Autodesk Fusion 360 part; units mm, degrees
note: some values were not read from the file. Set by a fixed rule: which face or edge a step refers to.
(part 2 of 2)
sketch "lid base (2)" plane through (0, 0, 0) normal (0, 0, 1) x (1, 0, 0) in component "lid, vented"
  line L0 (33.4, 49.8) -> (33.4, -1.75) construction
  line L1 (35, 49.8) -> (33.4, 49.8)
  line L2 (33.4, 55.6) -> (35, 55.6) construction
  line L3 (35, 55.6) -> (35, 66.15)
  line L4 (35, 49.8) -> (35, -1.75)
  line L5 (35, 49.8) -> (35, 55.6)
  line L6 (35, 66) -> (-9.2, 66)
  line L7 (-9.2, -1.6) -> (35, -1.6)
  line L8 (33.25, 49.8) -> (33.25, 0)
  line L9 (-7.45, 64.25) -> (33.25, 64.25)
  line L10 (33.25, 64.25) -> (33.25, 55.6)
  line L11 (-6.65, 0) -> (-6.65, 63.45)
  line L12 (32.45, 63.45) -> (32.45, 55.6)
  line L13 (35, 55.45) -> (32.45, 55.45)
  line L14 (32.45, 55.45) -> (32.45, 55.6)
  line L15 (33.25, 55.6) -> (33.25, 55.45)
  line L16 (33.4, -1.75) -> (-7.6, -1.75) construction
  line L17 (-7.6, 0) -> (33.4, 0)
  line L18 (-7.45, 0) -> (-7.45, -1.6)
  line L19 (33.25, 0) -> (33.25, -1.6)
  line L20 (31, 41) -> (33.4, 41)
  line L21 (35, 49.95) -> (32.45, 49.95)
  line L22 (32.45, 55.45) -> (32.45, 49.95)
  line L23 (32.45, 49.95) -> (32.45, 0)
  line L24 (32.45, 63.45) -> (32.45, 64.25)
  line L25 (-6.65, 63.45) -> (-6.65, 64.25)
  line L26 (33.25, 64.25) -> (33.25, 66)
  line L27 (33.25, 49.8) -> (33.25, 49.95)
  line L28 (-7.45, 64.25) -> (-7.45, 66)
  line L29 (-7.6, -1.75) -> (-9.2, -1.75) construction
  line L30 (-7.6, 66.15) -> (-9.2, 66.15) construction
  line L31 (-9.2, 55.6) -> (-9.2, 66.15)
  line L32 (-7.6, -1.75) -> (-7.6, 49.8) construction
  line L33 (33.4, 49.8) -> (33.4, -1.75) construction
  line L34 (33.4, 66.15) -> (33.4, 55.6) construction
  line L35 (35, -1.75) -> (33.4, -1.75) construction
  line L36 (35, 66.15) -> (33.4, 66.15) construction
  line L37 (0, 41) -> (-7.6, 41)
  line L38 (12.9, 64.25) -> (12.9, 0) construction
  line L39 (-9.2, 55.45) -> (-6.65, 55.45)
  line L40 (-9.2, 49.8) -> (-9.2, 55.6)
  line L41 (-9.2, 49.95) -> (-6.65, 49.95)
  line L42 (-7.45, 0) -> (-7.45, 49.95)
  line L43 (-7.45, 55.45) -> (-7.45, 64.25)
  line L44 (-9.2, -1.75) -> (-9.2, 49.8)
  line L45 (-7.6, 55.6) -> (-7.6, 66.15)
  dimension "d193_1" = 0.15
  dimension "d194_1" = 0.8
  dimension "d199_1" = 0.15
  dimension "d200_1" = 0.15
  dimension "d206_1" = 0.15
  dimension "d207_1" = 0.8
  dimension "d210_1" = 0.15
  constraint coincident L1.start L4.start
  constraint coincident L2.end L3.start
  constraint coincident L3 L6.start
  constraint coincident L4 L7.end
  constraint perpendicular L4 L7
  constraint coincident L5 L13.start
  constraint perpendicular L5 L13
  constraint perpendicular L13 L14
  constraint coincident L13 L15.end
  constraint perpendicular L13 L15
  constraint parallel L0 L8
  constraint collinear L8 L10
  constraint coincident L18.start L17
  constraint coincident L11.start L17
  constraint coincident L8.end L17
  constraint coincident L7 L18.end
  constraint perpendicular L7 L18
  constraint coincident L7 L19.end
  constraint perpendicular L7 L19
  constraint coincident L5 L21.start
  constraint perpendicular L14 L21
  constraint perpendicular L21 L22
  constraint coincident L17 L23.end
  constraint perpendicular L17 L23
  constraint coincident L9 L24.end
  constraint perpendicular L9 L24
  constraint coincident L9 L25.end
  constraint perpendicular L9 L25
  constraint coincident L6 L26.end
  constraint perpendicular L6 L26
  constraint coincident L21 L27.end
  constraint perpendicular L21 L27
  constraint coincident L6 L28.end
  constraint perpendicular L6 L28
  constraint midpoint L9 L38.start
  constraint midpoint L17 L38.end
  constraint perpendicular L17 L38
  constraint symmetric L1.start L38 L40.start
  constraint symmetric L2.end L38 L31.start
  constraint symmetric L13.start L38 L39.start
  constraint symmetric L13.end L38 L39.end
  constraint symmetric L21.start L38 L41.start
  constraint symmetric L21.end L38 L41.end
  constraint coincident L41 L42.end
  constraint coincident L39 L43.start
  constraint collinear L12 L24
  constraint perpendicular L39 L43
  measures "d193_1" distance of L7 L16
  measures "d194_1" distance of L11 L42
  measures "d199_1" distance of L0 L8
  measures "d200_1" distance of L2 L13
  measures "d206_1" distance of L1 L21
  measures "d207_1" distance of L8 L23
  measures "d210_1" distance of L6 L30
extrude "Extrude1'''" add sketch "lid base (2)" along normal blind 1.6 separate body makes body 3 in component "lid, vented"
extrude "Extrude2''" add sketch "lid base (2)" against normal blind 1.6 contours L5 L13 L21 L22 | L6 L9 L26 L28 | L9 L10 L12 L13 L14 L15 L24 | L8 L20 L21 L23 L27 | L9 L11 L25 L39 L43 | L11 L39 L40 L41 | L7 L17 L18 L19 | L11 L37 L41 L42 bodies 3 in component "lid, vented"
chamfer "Chamfer1''" distance 0.2 angle 45 1 edges at (35, 52.7, -1.6) on bodies 3 in component "lid, vented"
sketch "nubs (2)" plane through (0, 66, 0) normal (0, 1, 0) x (-1, 0, 0) in component "lid, vented"
  line L0 (-35, 0) -> (-33.25, 0)
  line L1 (-33.25, 0) -> (-33.25, -1.6)
  line L2 (-33.25, -1.6) -> (7.45, -1.6)
  line L3 (7.45, -1.6) -> (7.45, 0)
  line L4 (7.45, 0) -> (9.2, 0)
  line L5 (9.2, 0) -> (9.2, 1.6)
  line L6 (9.2, 1.6) -> (-35, 1.6)
  line L7 (-35, 1.6) -> (-35, 0)
  line L8 (-33.25, 0) -> (7.45, 0) construction
  line L9 (-27.65, -0.3) -> (-29.25, -0.3)
  line L10 (-29.25, -0.3) -> (-29.25, 0.3)
  line L11 (-29.25, 0.3) -> (-27.65, 0.3)
  line L12 (-27.65, 0.3) -> (-27.65, -0.3)
  line L13 (-27.65, -0.3) -> (-29.25, 0.3) construction
  line L14 (-29.25, -0.3) -> (-27.65, 0.3) construction
  line L15 (-12.9, 1.6) -> (-12.9, -1.6) construction
  line L16 (3.45, 0.3) -> (1.85, 0.3)
  line L17 (3.45, -0.3) -> (3.45, 0.3)
  line L18 (1.85, -0.3) -> (3.45, -0.3)
  line L19 (1.85, 0.3) -> (1.85, -0.3)
  point P0 (-28.45, 0)
  dimension "d213_1" = 1.6
  dimension "d214_1" = 0.6
  dimension "d215_1" = 4
  constraint coincident L0.end L1.start
  constraint coincident L3.end L4.start
  constraint horizontal L9
  constraint perpendicular L9 L10
  constraint parallel L9 L11
  constraint parallel L10 L12
  constraint coincident L13 P0
  constraint coincident L14 P0
  constraint coincident L8 P0
  constraint midpoint L6 L15.start
  constraint midpoint L2 L15.end
  constraint symmetric L9.start L15 L18.start
  constraint symmetric L9.end L15 L17.start
  constraint symmetric L10.end L15 L16.start
  constraint symmetric L11.end L15 L16.end
  measures "d213_1" distance of L10.end L11.end
  measures "d214_1" distance of L9.end L10.end
  measures "d215_1" distance of L1 L10
extrude "Extrude3''" add sketch "nubs (2)" along normal blind 0.35 contours L9 L10 L11 L12 | L16 L17 L18 L19 bodies 3 in component "lid, vented"
mirror "Mirror1''" about plane through (31.2, 32.2, -13) normal (0, 1, 0) of "Extrude3''" in component "lid, vented"
fillet "Fillet1''" radius 0.25 4 faces at (28.1833, 66.35, -0.1) (-2.3833, 66.35, -0.1) (28.1833, -1.95, -0.1) (-2.3833, -1.95, -0.1) on bodies 3 in component "lid, vented"
sketch "vent" plane through (0, 0, 0) normal (0, 0, -1) x (1, 0, 0) in component "lid, vented"
  line L0 (33.25, -49.95) -> (35, -49.95)
  line L1 (35, -49.95) -> (35, 1.6)
  line L2 (35, 1.6) -> (33.25, 1.6)
  line L3 (33.25, 1.6) -> (33.25, 0)
  line L4 (33.25, 0) -> (-7.45, 0)
  line L5 (-7.45, 0) -> (-7.45, 1.6)
  line L6 (-7.45, 1.6) -> (-9.2, 1.6)
  line L7 (-9.2, 1.6) -> (-9.2, -49.95)
  line L8 (-9.2, -49.95) -> (-7.45, -49.95)
  line L9 (-7.45, -49.95) -> (-7.45, -41)
  line L10 (-7.45, -41) -> (-6.65, -41)
  line L11 (-6.65, -41) -> (-6.65, -64.25)
  line L12 (-6.65, -64.25) -> (32.45, -64.25)
  line L13 (32.45, -64.25) -> (32.45, -41)
  line L14 (32.45, -41) -> (33.25, -41)
  line L15 (33.25, -41) -> (33.25, -49.95)
  line L16 (-6.65, -61.25) -> (21.85, -61.25) construction
  line L17 (21.85, -61.25) -> (21.85, -43.85) construction
  line L18 (21.85, -43.85) -> (-6.65, -43.85) construction
  line L19 (-6.65, -43.85) -> (-6.65, -61.25) construction
  line L20 (20.85, -44.85) -> (-5.65, -44.85) construction
  line L21 (-5.65, -44.85) -> (-5.65, -60.25) construction
  line L22 (-5.65, -60.25) -> (20.85, -60.25) construction
  line L23 (20.85, -60.25) -> (20.85, -44.85) construction
  line L24 (3.6, -44.85) -> (11.6, -60.25) construction
  line L25 (7.6, -60.25) -> (7.6, -44.85) construction
  line L26 (-12.4, -44.85) -> (-4.4, -60.25) construction
  line L27 (-8.4, -44.85) -> (-0.4, -60.25) construction
  line L28 (-4.4, -44.85) -> (3.6, -60.25) construction
  line L29 (-0.4, -44.85) -> (7.6, -60.25) construction
  line L30 (7.6, -44.85) -> (15.6, -60.25) construction
  line L31 (11.6, -44.85) -> (19.6, -60.25) construction
  line L32 (15.6, -44.85) -> (23.6, -60.25) construction
  line L33 (19.6, -44.85) -> (27.6, -60.25) construction
  line L34 (-5.9911, -58.9225) -> (-5.4787, -59.9089)
  arc A0 (-5.4787, -59.9089) -> (-4.0589, -59.1713) centre (-4.7688, -59.5401) ccw
  line L35 (-4.0589, -59.1713) -> (-4.5713, -58.1849)
  arc A1 (-4.5713, -58.1849) -> (-5.9911, -58.9225) centre (-5.2812, -58.5537) ccw
  line L36 (-5.65, -57.8438) -> (-4.4, -60.25) construction
  line L37 (-5.9911, -51.2225) -> (-1.4787, -59.9089)
  arc A2 (-1.4787, -59.9089) -> (-0.0589, -59.1713) centre (-0.7688, -59.5401) ccw
  line L38 (-0.0589, -59.1713) -> (-4.5713, -50.4849)
  arc A3 (-4.5713, -50.4849) -> (-5.9911, -51.2225) centre (-5.2812, -50.8537) ccw
  line L39 (-5.65, -50.1438) -> (-0.4, -60.25) construction
  line L40 (-4.7411, -45.9287) -> (2.5213, -59.9089)
  arc A4 (2.5213, -59.9089) -> (3.9411, -59.1713) centre (3.2312, -59.5401) ccw
  line L41 (3.9411, -59.1713) -> (-3.3213, -45.1911)
  arc A5 (-3.3213, -45.1911) -> (-4.7411, -45.9287) centre (-4.0312, -45.5599) ccw
  line L42 (-4.4, -44.85) -> (3.6, -60.25) construction
  line L43 (-0.7411, -45.9287) -> (6.5213, -59.9089)
  arc A6 (6.5213, -59.9089) -> (7.9411, -59.1713) centre (7.2312, -59.5401) ccw
  line L44 (7.9411, -59.1713) -> (0.6787, -45.1911)
  arc A7 (0.6787, -45.1911) -> (-0.7411, -45.9287) centre (-0.0312, -45.5599) ccw
  line L45 (-0.4, -44.85) -> (7.6, -60.25) construction
  line L46 (3.2589, -45.9287) -> (10.5213, -59.9089)
  arc A8 (10.5213, -59.9089) -> (11.9411, -59.1713) centre (11.2312, -59.5401) ccw
  line L47 (11.9411, -59.1713) -> (4.6787, -45.1911)
  arc A9 (4.6787, -45.1911) -> (3.2589, -45.9287) centre (3.9688, -45.5599) ccw
  line L48 (3.6, -44.85) -> (11.6, -60.25) construction
  line L49 (7.2589, -45.9287) -> (14.5213, -59.9089)
  arc A10 (14.5213, -59.9089) -> (15.9411, -59.1713) centre (15.2312, -59.5401) ccw
  line L50 (15.9411, -59.1713) -> (8.6787, -45.1911)
  arc A11 (8.6787, -45.1911) -> (7.2589, -45.9287) centre (7.9688, -45.5599) ccw
  line L51 (7.6, -44.85) -> (15.6, -60.25) construction
  line L52 (11.2589, -45.9287) -> (18.5213, -59.9089)
  arc A12 (18.5213, -59.9089) -> (19.9411, -59.1713) centre (19.2312, -59.5401) ccw
  line L53 (19.9411, -59.1713) -> (12.6787, -45.1911)
  arc A13 (12.6787, -45.1911) -> (11.2589, -45.9287) centre (11.9688, -45.5599) ccw
  line L54 (11.6, -44.85) -> (19.6, -60.25) construction
  line L55 (15.2589, -45.9287) -> (19.7713, -54.6151)
  arc A14 (19.7713, -54.6151) -> (21.1911, -53.8775) centre (20.4812, -54.2463) ccw
  line L56 (21.1911, -53.8775) -> (16.6787, -45.1911)
  arc A15 (16.6787, -45.1911) -> (15.2589, -45.9287) centre (15.9688, -45.5599) ccw
  line L57 (15.6, -44.85) -> (20.85, -54.9563) construction
  line L58 (19.2589, -45.9287) -> (19.7713, -46.9151)
  arc A16 (19.7713, -46.9151) -> (21.1911, -46.1775) centre (20.4812, -46.5463) ccw
  line L59 (21.1911, -46.1775) -> (20.6787, -45.1911)
  arc A17 (20.6787, -45.1911) -> (19.2589, -45.9287) centre (19.9688, -45.5599) ccw
  line L60 (19.6, -44.85) -> (20.85, -47.2562) construction
  point P0 (7.6, -52.55)
  dimension "d223" = 28.5
  dimension "d224" = 17.4
  dimension "d225" = 3
  dimension "d227" = -1
  dimension "d228" = 8
  dimension "d231" = 4
  dimension "d232" = 0
  dimension "d233" = 1.6
  dimension "d234" = 1.6
  dimension "d235" = 1.6
  dimension "d236" = 1.6
  dimension "d237" = 1.6
  dimension "d238" = 1.6
  dimension "d239" = 1.6
  dimension "d240" = 1.6
  dimension "d241" = 1.6
  constraint horizontal L16
  constraint vertical L17
  constraint horizontal L18
  constraint vertical L19
  constraint coincident L11 L16.start
  constraint coincident L20 L24.start
  constraint coincident L22 L24.end
  constraint midpoint L22 L25.start
  constraint midpoint L20 L25.end
  constraint midpoint L24 P0
  constraint coincident L25 P0
  constraint tangent L34 A0
  constraint tangent A0 L35
  constraint parallel L34 L35
  constraint tangent L35 A1
  constraint tangent L34 A1
  constraint midpoint A1 L36.start
  constraint midpoint L26.end A0
  constraint parallel L26 L36
  constraint coincident L21 L36.start
  constraint tangent L37 A2
  constraint tangent A2 L38
  constraint parallel L37 L38
  constraint tangent L38 A3
  constraint tangent L37 A3
  constraint midpoint A3 L39.start
  constraint midpoint L27.end A2
  constraint parallel L27 L39
  constraint coincident L21 L39.start
  constraint tangent L40 A4
  constraint tangent A4 L41
  constraint parallel L40 L41
  constraint tangent L41 A5
  constraint tangent L40 A5
  constraint midpoint L28.start A5
  constraint midpoint L28.end A4
  constraint tangent L43 A6
  constraint tangent A6 L44
  constraint parallel L43 L44
  constraint tangent L44 A7
  constraint tangent L43 A7
  constraint midpoint L29.start A7
  constraint midpoint L25.start A6
  constraint tangent L46 A8
  constraint tangent A8 L47
  constraint parallel L46 L47
  constraint tangent L47 A9
  constraint tangent L46 A9
  constraint midpoint L24.start A9
  constraint midpoint L24.end A8
  constraint tangent L49 A10
  constraint tangent A10 L50
  constraint parallel L49 L50
  constraint tangent L50 A11
  constraint tangent L49 A11
  constraint midpoint L25.end A11
  constraint midpoint L30.end A10
  constraint tangent L52 A12
  constraint tangent A12 L53
  constraint parallel L52 L53
  constraint tangent L53 A13
  constraint tangent L52 A13
  constraint midpoint L31.start A13
  constraint midpoint L31.end A12
  constraint tangent L55 A14
  constraint tangent A14 L56
  constraint parallel L55 L56
  constraint tangent L56 A15
  constraint tangent L55 A15
  constraint midpoint L32.start A15
  constraint midpoint A14 L57.end
  constraint coincident L23 L57.end
  constraint coincident L32 L57.end
  constraint tangent L58 A16
  constraint tangent A16 L59
  constraint parallel L58 L59
  constraint tangent L59 A17
  constraint tangent L58 A17
  constraint midpoint L33.start A17
  measures "d223" distance of L16.start L16.end
  measures "d224" distance of L16.start L18.end
  measures "d225" distance of L12 L16
  measures "d228" horizontal distance of L24.start L24.end
  measures "d233" diameter of A0
  measures "d234" diameter of A2
  measures "d235" diameter of A4
  measures "d236" diameter of A6
  measures "d237" diameter of A8
  measures "d238" diameter of A10
  measures "d239" diameter of A12
  measures "d240" diameter of A14
  measures "d241" diameter of A16
extrude "Extrude4'" cut sketch "vent" against normal through all contours L34 A0 L35 A1 | L37 A2 L38 A3 | L40 A4 L41 A5 | L43 A6 L44 A7 | L46 A8 L47 A9 | L49 A10 L50 A11 | L52 A12 L53 A13 | L55 A14 L56 A15 | L58 A16 L59 A17 bodies 3 in component "lid, vented"
component "case" placed x (1, 0, 0) y (0, 1, 0) z (0, 0, 1) at (0, 0, 1.6)
component "lid" placed x (1, 0, 0) y (0, 1, 0) z (0, 0, 1) at (0, 0, 17.6)
component "lid, vented" placed x (-1, 0, 0) y (0, 1, 0) z (0, 0, -1) at (75.7955, 0, 1.6)
equation "d121 = d119"
equation "d122 = d120"
equation "d197 = d193"
equation "d198 = d197"
equation "d199 = d198"
equation "d200 = d181"
equation "d206 = d200"
equation "d207 = d194"
equation "d199_1 = d198"
equation "d200_1 = d181"
equation "d206_1 = d200_1"
equation "d207_1 = d194_1"
